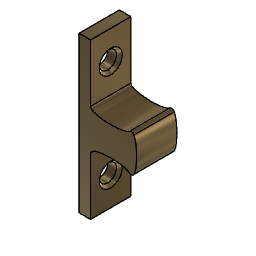
clip_connector_clip (Autodesk Fusion 360 design; units mm, degrees)
Autodesk Fusion 360 part; units mm, degrees
note: some values were not read from the file. Set by a fixed rule: which sketch regions a step uses.
sketch "Sketch1" plane through (0, 0, 0) normal (1, 0, 0) x (0, 1, 0)
  line L0 (0, 0) -> (7, 0)
  line L1 (7, 0) -> (7, 27)
  line L2 (7, 27) -> (0, 27)
  line L3 (0, 27) -> (0, 0)
  dimension "d1" = 7
  dimension "d2" = 27
  constraint horizontal L0
  constraint vertical L1
  constraint horizontal L2
  constraint vertical L3
  constraint coincident L0.start L3.end
  measures "d1" distance of L1.end L2.end
  measures "d2" distance of L0.end L1.end
extrude "Extrude1" add sketch "Sketch1" along normal blind 2
sketch "Sketch2" plane through (2, 0, 0) normal (1, 0, 0) x (0, 1, 0)
  line L0 (0, 27) -> (0, 0)
  line L1 (0, 0) -> (7, 0)
  line L2 (7, 0) -> (7, 27)
  line L3 (7, 27) -> (0, 27)
  line L4 (0, 17) -> (7, 17)
  line L5 (7, 17) -> (7, 10)
  line L6 (7, 10) -> (0, 10)
  line L7 (0, 10) -> (0, 17)
  circle A0 centre (3.5, 22) radius 1.5
  circle A1 centre (3.5, 5) radius 1.5
  dimension "d5" = 3.5
  dimension "d6" = 3.5
  dimension "d7" = 3
  dimension "d8" = 3
  dimension "d9" = 7
  dimension "d10" = 10
  dimension "d11" = 10
  dimension "d12" = 5
  dimension "d13" = 5
  dimension "d33" = 5
  dimension "d34" = 5
  constraint horizontal L4
  constraint vertical L5
  constraint horizontal L6
  constraint vertical L7
  constraint coincident L2 L5.end
  constraint coincident L0 L4.start
  measures "d5" distance of L0 A0.centre
  measures "d6" distance of L0 A1.centre
  measures "d7" diameter of A0
  measures "d8" diameter of A1
  measures "d9" distance of L4 L6
  measures "d10" distance of L3 L4
  measures "d11" distance of L1 L6
  measures "d12" distance of L3 A0.centre
  measures "d13" distance of L1 A1.centre
  measures "d33" distance of L4 A0.centre
  measures "d34" distance of L6 A1.centre
extrude "Extrude2" cut sketch "Sketch2" against normal blind 2 contours A0 | A1
chamfer "Chamfer1" distance 0.5 angle 45 2 edges at (2, 2.1015, 22.5424) (2, 2.1015, 5.5424)
extrude "Extrude3" add sketch "Sketch2" along normal blind 7 contours L0 L2 L4 L5 L6 L7
sketch "Sketch4" plane through (0, 0, 0) normal (0, -1, 0) x (1, 0, 0)
  line L0 (0, 27) -> (0, 0)
  line L1 (0, 0) -> (2, 0)
  line L2 (2, 0) -> (2, 10)
  line L3 (2, 10) -> (9, 10)
  line L4 (9, 10) -> (9, 17)
  line L5 (9, 17) -> (2, 17)
  line L6 (2, 17) -> (2, 27)
  line L7 (2, 27) -> (0, 27)
  ellipse E0 centre (9, 13.5) end of major axis (9, 17) minor radius 1
  line L8 (9, 10) -> (9, 17)
  line L9 (10, 13.5) -> (8, 13.5)
  dimension "d35" = 2
  constraint coincident L3.end E0
  constraint coincident L4.end E0
  constraint coincident E0 L9.start
  constraint coincident E0 L9.end
extrude "Extrude5" add sketch "Sketch4" against normal blind 7 contours L4 E0 L8 L9 | L4 E0 L8 L9 picked at (9.6303, 14.0297) picked at (9.2475, 11.5518)
sketch "Sketch5" plane through (0, 0, 0) normal (0, -1, 0) x (1, 0, 0)
  line L0 (0, 27) -> (0, 0)
  line L1 (0, 0) -> (2, 0)
  line L2 (2, 0) -> (2, 10)
  line L3 (2, 10) -> (9, 10)
  line L4 (9, 17) -> (2, 17)
  line L5 (2, 17) -> (2, 27)
  line L6 (2, 27) -> (0, 27)
  ellipse E0 centre (9, 13.5) end of major axis (9, 17) minor radius 1 (9, 10) -> (9, 17) ccw
  ellipse E1 centre (5.5, 17) end of major axis (9, 17) minor radius 1
  line L7 (2, 17) -> (9, 17)
  line L8 (5.5, 16) -> (5.5, 18)
  ellipse E2 centre (5.5, 10) end of major axis (9, 10) minor radius 1
  line L9 (2, 10) -> (9, 10)
  line L10 (5.5, 9) -> (5.5, 11)
  dimension "d36" = 2
  dimension "d37" = 2
  constraint coincident L4.end E1
  constraint coincident L4.start E1
  constraint coincident E1 L8.start
  constraint coincident E1 L8.end
  constraint coincident L4 E1.centre
  constraint coincident E2 L2.end
  constraint coincident L3.end E2
  constraint coincident E2 L10.start
  constraint coincident E2 L10.end
  constraint coincident L3 E2.centre
  constraint coincident L4.end L5.start
extrude "Extrude6" cut sketch "Sketch5" against normal blind 7 contours L4 E1 L7 L8 | L3 E2 L9 L10 | L4 E1 L7 L8 | L3 E2 L9 L10 picked at (3.5518, 16.7525) picked at (4.9703, 10.6303) picked at (6.0297, 16.3697) picked at (7.4482, 10.2475)
fillet "Fillet2" radius 0.5 2 edges at (9, 3.5, 17) (9, 3.5, 10)
equation "d5 = ( 7 / 2 ) * 1 mm"
equation "d6 = ( 7 / 2 ) * 1 mm"
equation "d10 = ( ( 27 - 7 ) / 2 ) * 1 mm"
equation "d12 = ( 10 / 2 ) * 1 mm"
equation "d13 = ( 10 / 2 ) * 1 mm"
named bodies: "Clip Connector Clip"
